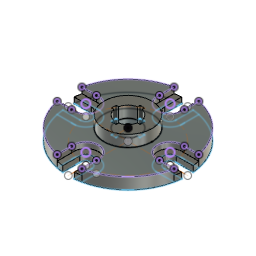
Model 4 (Autodesk Fusion 360 design; units mm, degrees)
Autodesk Fusion 360 part; units mm, degrees
sketch "Sketch8" plane through (0, 0, 0) normal (0, 0, 1) x (1, 0, 0)
  line L0 (0, 0) -> (0, 52.5) construction
  line L1 (0, 0) -> (0, -52.5) construction
  line L2 (0, 0) -> (52.5, 0) construction
  line L3 (0, 0) -> (-52.5, 0) construction
  line L4 (-35.3649, 10.8778) -> (-51.3607, 10.8778)
  line L5 (-35.3649, -10.8778) -> (-51.3607, -10.8778)
  line L6 (10.8778, 35.3649) -> (10.8778, 51.3607)
  line L7 (-10.8778, 35.3649) -> (-10.8778, 51.3607)
  line L8 (35.3649, 10.8778) -> (51.3607, 10.8778)
  line L9 (35.3649, -10.8778) -> (51.3607, -10.8778)
  line L10 (10.8778, -35.3649) -> (10.8778, -51.3607)
  line L11 (-10.8778, -35.3649) -> (-10.8778, -51.3607)
  line L12 (-4.9886, 36.6622) -> (-4.9886, 52.2625)
  line L13 (4.9886, 36.6622) -> (4.9886, 52.2625)
  line L14 (36.6622, 4.9886) -> (52.2625, 4.9886)
  line L15 (36.6622, -4.9886) -> (52.2625, -4.9886)
  line L16 (-4.9886, -36.6622) -> (-4.9886, -52.2625)
  line L17 (4.9886, -36.6622) -> (4.9886, -52.2625)
  line L18 (-36.6622, 4.9886) -> (-52.2625, 4.9886)
  line L19 (-36.6622, -4.9886) -> (-52.2625, -4.9886)
  arc A0 (-4.9886, 37.3378) -> (4.9886, 37.3378) centre (0, 37) ccw
  arc A1 (-10.8778, 38.6351) -> (10.8778, 38.6351) centre (0, 37) ccw
  arc A2 (35.3649, 10.8778) -> (36.6622, 4.9886) centre (0, 0) ccw construction
  arc A3 (38.6351, 10.8778) -> (38.6351, -10.8778) centre (37, 0) ccw
  arc A4 (37.3378, 4.9886) -> (37.3378, -4.9886) centre (37, 0) ccw
  arc A5 (10.8778, -38.6351) -> (-10.8778, -38.6351) centre (0, -37) ccw
  arc A6 (4.9886, -37.3378) -> (-4.9886, -37.3378) centre (0, -37) ccw
  arc A7 (-38.6351, -10.8778) -> (-38.6351, 10.8778) centre (-37, 0) ccw
  arc A8 (-37.3378, -4.9886) -> (-37.3378, 4.9886) centre (-37, 0) ccw
  arc A9 (-4.9886, 52.2625) -> (-52.2625, 4.9886) centre (0, 0) ccw
  arc A10 (52.2625, 4.9886) -> (4.9886, 52.2625) centre (0, 0) ccw
  arc A11 (-52.2625, -4.9886) -> (-4.9886, -52.2625) centre (0, 0) ccw
  arc A12 (4.9886, -52.2625) -> (52.2625, -4.9886) centre (0, 0) ccw
  dimension "d65" = 105
  dimension "d66" = 74
  dimension "d67" = 22
  dimension "d68" = 10
  constraint coincident L0.start L1.start
  constraint vertical L0
  constraint coincident L1.end A9
  constraint coincident L2.end A9
  constraint coincident L3.end A9
  constraint coincident L0 A0.centre
  constraint coincident A0.centre A2
  constraint concentric A0 A1
  constraint coincident L4.start A2
  constraint coincident L4.start A7
  constraint coincident L4.end A9
  constraint horizontal L4
  constraint coincident L5.start A7
  constraint coincident L5.start A2
  constraint coincident L5.end A9
  constraint parallel L4 L5
  constraint coincident L6.start A1
  constraint coincident L6.start A2
  constraint coincident L6.end A9
  constraint perpendicular L5 L6
  constraint coincident L7.start A1
  constraint coincident L7.start A2
  constraint coincident L7.end A9
  constraint parallel L6 L7
  constraint coincident L8.start A3
  constraint coincident L8.end A9
  constraint perpendicular L7 L8
  constraint coincident L9.start A3
  constraint coincident L9.start A2
  constraint coincident L9.end A9
  constraint parallel L8 L9
  constraint coincident L10.start A5
  constraint coincident L10.start A2
  constraint coincident L10.end A9
  constraint perpendicular L9 L10
  constraint coincident L11.start A5
  constraint coincident L11.start A2
  constraint coincident L11.end A9
  constraint parallel L10 L11
  constraint coincident L12.start A0
  constraint coincident L12.start A2
  constraint vertical L12
  constraint coincident L13.start A0
  constraint coincident L13.start A2
  constraint parallel L12 L13
  constraint coincident L14.start A4
  constraint coincident L14.end A9
  constraint perpendicular L13 L14
  constraint coincident L15.start A4
  constraint coincident L15.start A2
  constraint coincident L15.end A9
  constraint parallel L14 L15
  constraint coincident L16.start A6
  constraint coincident L16.start A2
  constraint coincident L16.end A9
  constraint perpendicular L15 L16
  constraint coincident L17.start A2
  constraint coincident L17.start A6
  constraint coincident L17.end A9
  constraint parallel L16 L17
  constraint coincident L18.start A8
  constraint coincident L18.start A2
  constraint perpendicular L17 L18
  constraint coincident L19.start A8
  constraint coincident L19.start A2
  constraint coincident L19.end A9
  constraint parallel L18 L19
  constraint coincident L13 A0.end
  constraint coincident L12 A0.start
  constraint coincident L7 A1.start
  constraint coincident L6 A1.end
  constraint coincident L14 A4.start
  constraint coincident L15 A4.end
  constraint coincident L8 A3.start
  constraint coincident L9 A3.end
  constraint coincident L10 A5.start
  constraint coincident L11 A5.end
  constraint coincident L17 A6.start
  constraint coincident L16 A6.end
  constraint coincident L4 A7.end
  constraint coincident L5 A7.start
  constraint coincident L19 A8.start
  constraint coincident L18 A8.end
  measures "d65" diameter of A9
  measures "d66" diameter of A2
  measures "d67" diameter of A1
  measures "d68" diameter of A0
extrude "Extrude9" add sketch "Sketch8" along normal blind 10 contours L4 L5 L6 L7 L8 L9 L10 L11 A1 A3 A5 A7 A9 A10 A11 A12 makes body 1
extrude "Extrude10" add sketch "Sketch8" along normal blind 5 separate body contours L4 L5 L18 L19 A7 A8 A9 A11 | L6 L7 L12 L13 A0 A1 A9 A10 | L10 L11 L16 L17 A5 A6 A11 A12 | L8 L9 L14 L15 A3 A4 A10 A12 makes body 2 at (41.3545, 8.9147, 0) makes body 3 at (8.9147, -41.3545, 0) makes body 4 at (-8.9147, 41.3545, 5) makes body 5 at (-41.3545, -8.9147, 0)
sketch "Sketch13" plane through (0, 0, 10) normal (0, 0, 1) x (1, 0, 0)
  circle A0 centre (0, 0) radius 21
  line L0 (2, -12.5) -> (-2, -12.5)
  line L1 (0, 0) -> (0, -12.5) construction
  line L2 (2, -10.3078) -> (2, -12.5)
  line L3 (-2, -10.3078) -> (-2, -12.5)
  line L4 (12.5, 2) -> (12.5, -2)
  line L5 (10.3078, 2) -> (12.5, 2)
  line L6 (10.3078, -2) -> (12.5, -2)
  line L7 (-2, 12.5) -> (2, 12.5)
  line L8 (-2, 10.3078) -> (-2, 12.5)
  line L9 (2, 10.3078) -> (2, 12.5)
  line L10 (-12.5, -2) -> (-12.5, 2)
  line L11 (-10.3078, -2) -> (-12.5, -2)
  line L12 (-10.3078, 2) -> (-12.5, 2)
  arc A1 (-10.3078, -2) -> (-2, -10.3078) centre (0, 0) ccw
  arc A2 (2, -10.3078) -> (10.3078, -2) centre (0, 0) ccw
  arc A3 (10.3078, 2) -> (2, 10.3078) centre (0, 0) ccw
  arc A4 (-2, 10.3078) -> (-10.3078, 2) centre (0, 0) ccw
  arc A5 (10.8778, -38.6351) -> (-10.8778, -38.6351) centre (0, -37) ccw
  line L13 (10.8778, -38.6351) -> (10.8778, -51.3607)
  arc A6 (10.8778, -51.3607) -> (51.3607, -10.8778) centre (0, 0) ccw
  line L14 (51.3607, -10.8778) -> (38.6351, -10.8778)
  arc A7 (38.6351, 10.8778) -> (38.6351, -10.8778) centre (37, 0) ccw
  line L15 (38.6351, 10.8778) -> (51.3607, 10.8778)
  arc A8 (51.3607, 10.8778) -> (10.8778, 51.3607) centre (0, 0) ccw
  line L16 (10.8778, 51.3607) -> (10.8778, 38.6351)
  arc A9 (-10.8778, 38.6351) -> (10.8778, 38.6351) centre (0, 37) ccw
  line L17 (-10.8778, 38.6351) -> (-10.8778, 51.3607)
  arc A10 (-10.8778, 51.3607) -> (-51.3607, 10.8778) centre (0, 0) ccw
  line L18 (-51.3607, 10.8778) -> (-38.6351, 10.8778)
  arc A11 (-38.6351, -10.8778) -> (-38.6351, 10.8778) centre (-37, 0) ccw
  line L19 (-38.6351, -10.8778) -> (-51.3607, -10.8778)
  arc A12 (-51.3607, -10.8778) -> (-10.8778, -51.3607) centre (0, 0) ccw
  line L20 (-10.8778, -51.3607) -> (-10.8778, -38.6351)
  dimension "d83" = 42
  dimension "d84" = 21
  dimension "d90" = 360
  dimension "d95" = 4
  dimension "d97" = 2
  constraint coincident A0.centre L1.start
  constraint perpendicular L0 L2
  constraint perpendicular L0 L3
  constraint coincident L0 L1.end
  constraint concentric A1 A2
  constraint concentric A2 A3
  constraint concentric A3 A4
  measures "d83" diameter of A0
  measures "d84" diameter of A2
  measures "d95" distance of L7.start L7.end
  measures "d97" distance of L9 A0.centre
extrude "Extrude11" add sketch "Sketch13" along normal blind 10 contours A0 bodies 1
extrude "Extrude12" cut sketch "Sketch13" against normal blind 15 contours L0 L2 L3 L4 L5 L6 L7 L8 L9 L10 L11 L12 A1 A2 A3 A4 bodies 1
